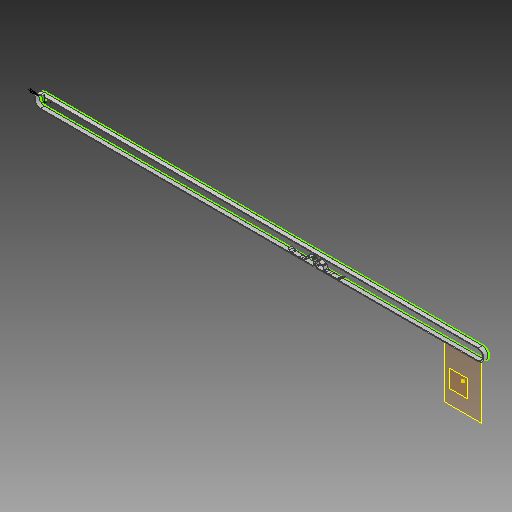
# Autodesk Inventor part: XBELT
Saved by Autodesk Inventor 2018 (Build 220112000, 112)
## iProperties
Created: 2016-07-22
Part Number: XBELT
Material: Generic
Document SubType Name: Modeling
Designer: User
Density: 1 g/cm^3
Appearance: Default
Mass: 6.77327 g
Surface Area: 158.043 cm^2
Volume: 6.77327 cm^3
Author: User
Autodesk Inventor part; units mm, degrees
ref_plane "YZ Plane" through (0, 0, 0) normal (1, 0, 0) x (0, 1, 0)
ref_plane "XZ Plane" through (0, 0, 0) normal (0, 1, 0) x (-1, 0, 0)
ref_plane "XY Plane" through (0, 0, 0) normal (0, 0, 1) x (1, 0, 0)
ref_plane "Work Plane1" through (0, 0, 0) normal (0, 0, 1) x (1, 0, 0)
sketch "Sketch1" plane through (0, 0, 0) normal (0, 0, 1) x (1, 0, 0)
  arc A0 (24.6543, 36.9901) -> (24.6581, 49.8888) centre (24.6562, 43.4394) ccw
  arc A1 (-523.0049, 50.5993) -> (-523.009, 36.5993) centre (-523.014, 43.5993) ccw
  line L0 (-523.009, 36.5993) -> (24.8958, 36.9945)
  line L1 (24.9813, 49.8806) -> (-523.0049, 50.5993)
  line L2 (-523.0083, 35.5993) -> (24.9141, 35.9946)
  arc A2 (24.655, 35.9901) -> (24.666, 50.8888) centre (24.6562, 43.4394) ccw
  arc A3 (-523.0035, 51.5993) -> (-523.0083, 35.5993) centre (-523.014, 43.5993) ccw
  line L3 (-523.0035, 51.5993) -> (25.0062, 50.8806)
  point P0 (0, 0)
  dimension "d0" = 1
  constraints: 12 point on circle, 9 end point, 4 centre point
  measures "d0" radial gap between concentric circles of A1 A3
ref_plane "Work Plane2" through (0, 0, 6) normal (0, 0, 1) x (1, 0, 0)
sketch "Sketch2" plane through (0, 0, 6) normal (0, 0, 1) x (1, 0, 0)
  line L0 (-523.0049, 50.5993) -> (24.9813, 49.8806)
  arc A0 (26.1347, 37.1513) -> (24.9813, 49.8806) centre (24.6937, 43.4377) ccw
  arc A1 (-523.0049, 50.5993) -> (-523.0019, 36.5993) centre (-523.0069, 43.5993) ccw
  line L1 (-523.0501, 35.5895) -> (-182.2036, 35.8354)
  arc A2 (24.8737, 35.9804) -> (24.9644, 50.8708) centre (24.674, 43.4271) ccw
  line L2 (24.9644, 50.8708) -> (-523.0453, 51.5895)
  arc A3 (-523.0453, 51.5895) -> (-523.0501, 35.5895) centre (-523.0477, 43.5895) ccw
  line L3 (26.1347, 37.1513) -> (-177.3524, 36.8243)
  line L4 (26.1347, 37.1513) -> (-177.3524, 36.8243)
  line L5 (-177.55, 35.8233) -> (24.8737, 35.9804)
  line L6 (-182.3943, 36.845) -> (-523.0019, 36.5993)
  line L7 (-182.3943, 36.845) -> (-523.0019, 36.5993)
  line L8 (-182.3943, 36.845) -> (-523.009, 36.5993)
  arc A4 (-175.5981, 44.0056) -> (-177.8793, 42.0255) centre (-175.8793, 42.0255) ccw projected
  line L9 (-177.8793, 42.0255) -> (-177.8793, 38.1674) projected
  line L10 (-168.9783, 38.1674) -> (-177.8793, 38.1674) projected
  arc A5 (-168.9783, 38.1674) -> (-168.8741, 38.8755) centre (-169.5783, 38.6174) ccw projected
  line L11 (-168.8741, 38.8755) -> (-169.5014, 41.4937) projected
  arc A6 (-169.5014, 41.4937) -> (-170.852, 42.9373) centre (-171.4464, 41.0276) ccw projected
  arc A7 (-170.852, 42.9373) -> (-175.5981, 44.0056) centre (-179.8602, 13.9956) ccw projected
  arc A8 (-181.8793, 42.02) -> (-184.1633, 43.9998) centre (-183.8793, 42.02) ccw projected
  arc A9 (-184.1633, 43.9998) -> (-188.8754, 42.9351) centre (-179.8602, 13.9956) ccw projected
  arc A10 (-188.8754, 42.9351) -> (-190.223, 41.5019) centre (-188.2805, 41.0256) ccw projected
  line L12 (-190.223, 41.5019) -> (-190.8453, 38.9643) projected
  arc A11 (-190.8453, 38.9643) -> (-190.7804, 38.1674) centre (-190.1804, 38.6174) ccw projected
  line L13 (-181.8793, 38.1674) -> (-190.7804, 38.1674) projected
  line L14 (-181.8793, 42.02) -> (-181.8793, 38.1674) projected
  line L15 (-177.3524, 36.8243) -> (-177.8746, 37.7286)
  line L16 (-177.8746, 37.7286) -> (-178.2063, 38.5555)
  line L17 (-178.2063, 38.5555) -> (-178.2078, 40.6305)
  line L18 (-178.2078, 40.6305) -> (-178.209, 42.3362)
  line L19 (-178.209, 42.3362) -> (-177.737, 43.3845)
  line L20 (-177.737, 43.3845) -> (-177.1904, 43.8398)
  line L21 (-177.1904, 43.8398) -> (-176.2125, 44.2321)
  line L22 (-176.2125, 44.2321) -> (-175.2227, 44.2328)
  line L23 (-175.2227, 44.2328) -> (-170.4599, 42.9351)
  line L24 (-170.4599, 42.9351) -> (-169.9859, 42.5772)
  line L25 (-169.9859, 42.5772) -> (-169.4819, 41.9721)
  line L26 (-169.4819, 41.9721) -> (-168.629, 38.4129)
  line L27 (-168.629, 38.4129) -> (-167.76, 37.7567)
  line L28 (-167.76, 37.7567) -> (-165.9159, 37.2737)
  line L29 (-165.9159, 37.2737) -> (-163.1275, 36.9945)
  line L30 (-163.1275, 36.9945) -> (-160.3695, 36.9965)
  line L31 (-160.3695, 36.9965) -> (-151.627, 37.2737)
  line L32 (-151.627, 37.2737) -> (-150.5918, 37.5217)
  line L33 (-150.5918, 37.5217) -> (-148.0211, 38.5527)
  line L34 (-148.0211, 38.5527) -> (-146.3842, 39.9163)
  line L35 (-146.3842, 39.9163) -> (-146.6143, 40.1925)
  line L36 (-146.6143, 40.1925) -> (-148.2512, 38.8289)
  line L37 (-148.2512, 38.8289) -> (-150.6724, 37.8579)
  line L38 (-150.6724, 37.8579) -> (-151.8853, 37.5672)
  line L39 (-151.8853, 37.5672) -> (-160.472, 37.295)
  line L40 (-160.472, 37.295) -> (-163.1702, 37.4311)
  line L41 (-163.1702, 37.4311) -> (-165.8102, 37.5643)
  line L42 (-165.8102, 37.5643) -> (-167.6157, 38.0372)
  line L43 (-167.6157, 38.0372) -> (-168.2752, 38.8289)
  line L44 (-168.2752, 38.8289) -> (-169.2827, 42.138)
  line L45 (-169.2827, 42.138) -> (-169.6866, 42.8265)
  line L46 (-169.6866, 42.8265) -> (-170.4021, 43.1486)
  line L47 (-170.4021, 43.1486) -> (-175.2236, 44.4623)
  line L48 (-175.2236, 44.4623) -> (-175.9859, 44.5387)
  line L49 (-175.9859, 44.5387) -> (-176.8242, 44.3378)
  line L50 (-176.8242, 44.3378) -> (-177.6272, 43.8055)
  line L51 (-177.6272, 43.8055) -> (-178.135, 43.3825)
  line L52 (-178.135, 43.3825) -> (-178.4245, 42.5752)
  line L53 (-178.4245, 42.5752) -> (-178.6341, 40.4815)
  line L54 (-178.6341, 40.4815) -> (-178.4776, 38.0352)
  line L55 (-178.4776, 38.0352) -> (-177.55, 35.8233)
  line L56 (-177.8793, 40.4835) -> (-181.8793, 40.4835)
  line L57 (-179.8793, 40.4835) -> (-179.8793, 39.2603)
  arc A12 (-181.8793, 42.0255) -> (-184.1606, 44.0056) centre (-183.8793, 42.0255) ccw
  line L58 (-181.8793, 42.0255) -> (-181.8793, 38.1674)
  line L59 (-190.7804, 38.1674) -> (-181.8793, 38.1674)
  arc A13 (-190.8846, 38.8755) -> (-190.7804, 38.1674) centre (-190.1804, 38.6174) ccw
  line L60 (-190.8846, 38.8755) -> (-190.2572, 41.4937)
  arc A14 (-188.9067, 42.9373) -> (-190.2572, 41.4937) centre (-188.3123, 41.0276) ccw
  arc A15 (-184.1606, 44.0056) -> (-188.9067, 42.9373) centre (-179.8985, 13.9956) ccw
  line L61 (-182.3943, 36.845) -> (-181.8841, 37.7286)
  line L62 (-181.8841, 37.7286) -> (-181.5524, 38.5555)
  line L63 (-181.5524, 38.5555) -> (-181.5509, 40.6305)
  line L64 (-181.5509, 40.6305) -> (-181.5497, 42.3362)
  line L65 (-181.5497, 42.3362) -> (-182.0217, 43.3845)
  line L66 (-182.0217, 43.3845) -> (-182.5683, 43.8398)
  line L67 (-182.5683, 43.8398) -> (-183.5462, 44.2321)
  line L68 (-183.5462, 44.2321) -> (-184.536, 44.2328)
  line L69 (-184.536, 44.2328) -> (-189.2987, 42.9351)
  line L70 (-189.2987, 42.9351) -> (-189.7728, 42.5772)
  line L71 (-189.7728, 42.5772) -> (-190.2768, 41.9721)
  line L72 (-190.2768, 41.9721) -> (-191.1297, 38.4129)
  line L73 (-191.1297, 38.4129) -> (-191.9987, 37.7567)
  line L74 (-191.9987, 37.7567) -> (-193.8428, 37.2737)
  line L75 (-193.8428, 37.2737) -> (-196.6311, 36.9945)
  line L76 (-196.6311, 36.9945) -> (-199.3891, 36.9965)
  line L77 (-199.3891, 36.9965) -> (-208.1317, 37.2737)
  line L78 (-208.1317, 37.2737) -> (-209.1668, 37.5217)
  line L79 (-209.1668, 37.5217) -> (-211.7376, 38.5527)
  line L80 (-211.7376, 38.5527) -> (-213.3745, 39.9163)
  line L81 (-213.3745, 39.9163) -> (-213.1444, 40.1925)
  line L82 (-213.1444, 40.1925) -> (-211.5075, 38.8289)
  line L83 (-211.5075, 38.8289) -> (-209.0863, 37.8579)
  line L84 (-209.0863, 37.8579) -> (-207.8734, 37.5672)
  line L85 (-207.8734, 37.5672) -> (-199.2867, 37.295)
  line L86 (-199.2867, 37.295) -> (-196.5885, 37.4311)
  line L87 (-196.5885, 37.4311) -> (-193.9485, 37.5643)
  line L88 (-193.9485, 37.5643) -> (-192.143, 38.0372)
  line L89 (-192.143, 38.0372) -> (-191.4835, 38.8289)
  line L90 (-191.4835, 38.8289) -> (-190.476, 42.138)
  line L91 (-190.476, 42.138) -> (-190.0721, 42.8265)
  line L92 (-190.0721, 42.8265) -> (-189.3566, 43.1486)
  line L93 (-189.3566, 43.1486) -> (-184.5351, 44.4623)
  line L94 (-184.5351, 44.4623) -> (-183.7728, 44.5387)
  line L95 (-183.7728, 44.5387) -> (-182.9345, 44.3378)
  line L96 (-182.9345, 44.3378) -> (-182.1314, 43.8055)
  line L97 (-182.1314, 43.8055) -> (-181.6237, 43.3825)
  line L98 (-181.6237, 43.3825) -> (-181.3342, 42.5752)
  line L99 (-181.3342, 42.5752) -> (-181.1246, 40.4815)
  line L100 (-181.1246, 40.4815) -> (-181.2811, 38.0352)
  line L101 (-181.2811, 38.0352) -> (-182.2036, 35.8354)
  point P0 (-182.2087, 35.8233)
  point P1 (-182.4063, 36.8243)
  constraints: 187 end point, 51 symmetric about line, 15 point on line, 12 perpendicular, 10 parallel, 8 point on circle, 7 centre point, 1 midpoint, 4 other
extrude "Extrusion2" add sketch "Sketch2" against normal blind 5 contours A1 L6 L61 L62 L63 L56 L100 L101 L1 A3 L2 A2 L5 L55 L54 L17 L16 L15 L3 A0 L0 | L56 L53 L52 L51 L50 L49 L48 L47 L46 L45 L44 L43 L42 L41 L40 L39 L38 L37 L36 L35 L34 L33 L32 L31 L30 L29 L28 L27 L26 L25 L24 L23 L22 L21 L20 L19 L18 L17 | L63 L64 L65 L66 L67 L68 L69 L70 L71 L72 L73 L74 L75 L76 L77 L78 L79 L80 L81 L82 L83 L84 L85 L86 L87 L88 L89 L90 L91 L92 L93 L94 L95 L96 L97 L98 L99 L56
body "Solid2"
